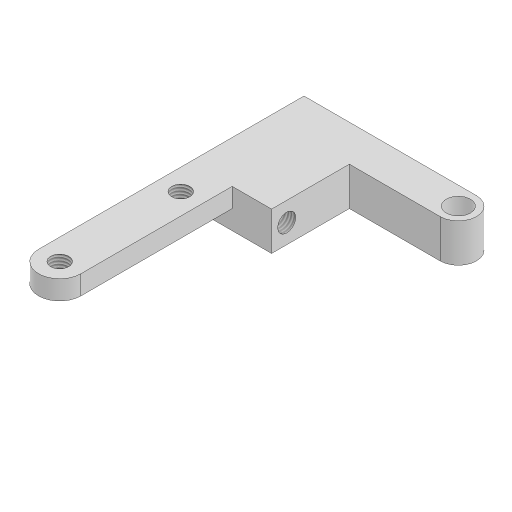
# Autodesk Inventor part: mgn9SlideBearingHolderWithCableManegment
Saved by Autodesk Inventor 2023 (Build 270158000, 158)
## iProperties
Created: 2022-11-03
Part Number: mgn9SlideBearingHolderWithCableManegment
Material: Generic
Document SubType Name: Modeling
Designer: deli
Density: 1 g/cm^3
Appearance: Default
Author: deli
Autodesk Inventor part; units mm, degrees
ref_plane "YZ Plane" through (0, 0, 0) normal (1, 0, 0) x (0, 1, 0)
ref_plane "XZ Plane" through (0, 0, 0) normal (0, 1, 0) x (-1, 0, 0)
ref_plane "XY Plane" through (0, 0, 0) normal (0, 0, 1) x (1, 0, 0)
sketch "Sketch1" plane through (0, 0, 0) normal (0, 1, 0) x (-1, 0, 0)
  circle A0 centre (7.2873, 50.1345) radius 1.5
  circle A1 centre (7.2873, 30.1345) radius 1.5
  arc A2 (10.7873, 50.1345) -> (3.7873, 50.1345) centre (7.2873, 50.1345) ccw
  line L0 (10.7873, 50.1345) -> (10.7873, 6.2845)
  line L1 (10.7873, 6.2845) -> (5.6806, 6.2845)
  line L2 (3.7873, 25.1345) -> (3.7873, 50.1345)
  line L3 (5.6806, 6.2845) -> (-2.7127, 6.2845)
  line L4 (-2.7127, 6.2845) -> (-2.7127, 25.1345)
  line L5 (-2.7127, 25.1345) -> (3.7873, 25.1345)
  point P0 (0, 0)
  dimension "d0" = 3
  dimension "d1" = 2
  dimension "d2" = 20
  dimension "d3" = 23.85
  dimension "d19" = 18.85
  dimension "d20" = 10
  dimension "d27" = 3.5
  constraints: 12 end point, 3 centre point, 2 perpendicular, 2 point on circle, 2 tangent, 1 coincident, 1 equal radius, 1 horizontal, 1 parallel, 1 vertical
  measures "d0" diameter of A0
  measures "d1" radial gap between concentric circles of A2 A0
  measures "d2" distance of A0.centre A1.centre
  measures "d3" distance from line of L1 A1.centre
  measures "d19" distance between parallel lines of L5 L3
  measures "d20" distance from line of A1.centre L4
  measures "d27" distance from line of L0 A1.centre
extrude "Extrusion1" add sketch "Sketch1" along normal blind 3.175
sketch "Sketch2" plane through (0, 3.175, 0) normal (0, 1, 0) x (1, 0, 0)
  line L0 (-10.7873, -6.2845) -> (2.7127, -6.2845)
  line L1 (2.7127, -6.2845) -> (2.7127, -25.1345)
  line L2 (2.7127, -25.1345) -> (-10.7873, -25.1345)
  line L3 (-10.7873, -25.1345) -> (-10.7873, -6.2845)
  point P0 (0, 0)
  point P1 (2.7127, -25.1345)
  constraints: 8 end point, 2 coincident, 2 parallel, 1 horizontal, 1 perpendicular
extrude "Extrusion2" add sketch "Sketch2" against normal blind 6.35
thread "Thread1" size "M3x0.5" class "6H" standard "ANSI Metric M Profile" full length
thread "Thread3" size "M3x0.5" class "6H" standard "ANSI Metric M Profile" full length
sketch "Sketch4" plane through (2.7127, 0, 25.1345) normal (1, 0, 0) x (0, 0, 1)
  line L0 (0, 0) -> (25, 0) projected
  circle A0 centre (-2.5, 0) radius 1.5
  line L1 (0, 0) -> (0, 3.175) construction
  line L2 (-18.85, -3.175) -> (25, -3.175) construction
  point P0 (-25.1345, 0)
  dimension "d26" = 3
  dimension "d28" = 3.175
  dimension "d29" = 1
  constraints: 1 centre point, 1 coincident
  measures "d26" diameter of A0
  measures "d28" distance from line of L2 A0.centre
  measures "d29" distance edge to line of A0 L1
extrude "Extrusion4" cut sketch "Sketch4" against normal blind 8
thread "Thread4" size "M3x0.5" class "6H" standard "ANSI Metric M Profile" full length
sketch "Sketch6" plane through (0, 3.175, 0) normal (0, 1, 0) x (1, 0, 0)
  line L0 (2.7127, -25.1345) -> (2.7127, -6.2845) projected
  line L1 (2.7127, -6.2845) -> (17.7127, -6.2845)
  line L2 (2.7127, -12.2845) -> (17.7127, -12.2845)
  arc A0 (17.7127, -12.2845) -> (17.7127, -6.2845) centre (17.7127, -9.2845) ccw
  circle A1 centre (17.7127, -9.2845) radius 2
  point P0 (0, 0)
  dimension "d30" = 6
  dimension "d31" = 4
  dimension "d32" = 15
  constraints: 4 end point, 2 centre point, 2 horizontal, 2 point on circle, 2 tangent, 1 coincident, 1 point on line
  measures "d30" diameter of A0
  measures "d31" diameter of A1
  measures "d32" distance of L2.start L2.end
extrude "Extrusion5" add sketch "Sketch6" against normal blind 6.35
equation "\"d27\" = d1 + 0.5 * d0"
body "Solid1"
